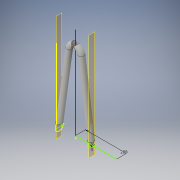
# Autodesk Inventor part: upper_arm_001
Saved by Autodesk Inventor 2016 SP1 (Build 200210100, 210)
## iProperties
Created: 2016-06-15
Part Number: upper_arm_001
Material: Generic
Document SubType Name: Modeling
Designer: asvsf
Density: 1 g/cm^3
Appearance: Default
Author: asvsf
Autodesk Inventor part; units mm, degrees
ref_plane "XZ Plane" through (0, 0, 0) normal (0, 1, 0) x (-1, 0, 0)
ref_plane "XY Plane" through (0, 0, 0) normal (0, 0, 1) x (1, 0, 0)
sketch "Sketch1" plane through (0, 0, 0) normal (0, 1, 0) x (-1, 0, 0)
  line L0 (-80, 0) -> (-30, 356.5109)
  line L1 (0, 0) -> (0, 520.9194)
  line L2 (80, 0) -> (30, 356.5109)
  arc A0 (30, 356.5109) -> (-30, 356.5109) centre (0, 352.3034) ccw
  dimension "d66" = 360
  dimension "d67" = 80
  dimension "d68" = 60
  dimension "d71" = 80
  constraints: 6 end point, 2 point on circle, 2 symmetric about line, 2 tangent, 1 centre point, 1 vertical
  measures "d66" distance of L0.start L0.end
  measures "d67" distance of L1.start L0.start
  measures "d68" distance of L2.end L0.end
  measures "d71" distance of L1.start L2.start
sketch "Sketch8" plane through (0, 0, 0) normal (0, 1, 0) x (-1, 0, 0)
  line L0 (0, 0) -> (0, 447.7409)
  constraints: 2 end point, 1 vertical
sketch "Sketch15" plane through (0, 0, 0) normal (1, 0, 0) x (0, 1, 0)
  line L0 (0, 0) -> (0, 447.7409) projected
  ellipse E0 centre (0, 0) end of major axis (13, 0) minor radius 2.8889 projected
  circle A0 centre (0, -17.1111) radius 20
  line L1 (0, 2.8889) -> (0, 11.2074)
  line L2 (0, 2.8889) -> (0, 15.4225)
  dimension "d60" = 40
  constraints: 4 end point, 2 coincident, 2 point on line, 2 vertical alignment, 1 vertical, 3 other
ref_plane "Work Plane6" through (80, 0, 0) normal (-0.1388889, 0, 0.990308) x (0, -1, 0)
sketch "Sketch16" plane through (80, 0, 0) normal (-0.1388889, 0, 0.990308) x (0, -1, 0)
  circle A0 centre (0, 0) radius 13
  point P0 (0, -79.2246)
  dimension "d72" = 26
  constraints: 1 centre point
  measures "d72" diameter of A0
sweep "Sweep5" add profiles "Sketch16" path "Sketch1" path curves L0 A0 L2
extrude "Extrusion8" [suppressed]
sketch "Sketch17" plane through (0, 0, 0) normal (0, 0, 1) x (1, 0, 0)
  line L0 (-30, -13) -> (30, -13) projected
  circle A0 centre (0, 0) radius 14
  dimension "d81" = 28
  constraints: 1 centre point
  measures "d81" diameter of A0
extrude "Extrusion9" cut sketch "Sketch17" along normal through all
sketch "Sketch18" plane through (0, 0, 0) normal (1, 0, 0) x (0, 1, 0)
  circle A0 centre (0, 0) radius 20
  ellipse E0 centre (0, 0) end of major axis (13, 0) minor radius 1.8056 projected
  dimension "d86" = 40
  constraints: 1 centre point, 1 coincident, 1 other
  measures "d86" diameter of A0
extrude "Extrusion10" cut sketch "Sketch18" along normal through all both and the other way through all contours A0 | E0
sketch "Sketch20" plane through (0, 0, 0) normal (0, 0, 1) x (1, 0, 0)
  line L0 (0, 0) -> (200, 0)
  point P0 (80, 0)
  dimension "d94" = 200
  constraints: 2 end point, 1 horizontal
  measures "d94" distance of L0.start L0.end
ref_plane "Work Plane7" through (80, 0, 0) normal (1, 0, 0) x (0, 1, 0)
sketch "Sketch22" plane through (80, 0, 0) normal (1, 0, 0) x (0, 1, 0)
  line L0 (0, 0) -> (0, -24.8938)
  constraints: 2 end point, 1 vertical
ref_plane "Work Plane8" through (-80, 0, 0) normal (1, 0, 0) x (0, 1, 0)
sketch "Sketch23" plane through (-80, 0, 0) normal (1, 0, 0) x (0, 1, 0)
  line L0 (-13, 356.5109) -> (-13, 15.1987) projected
  line L1 (-13, -2.9958) -> (30.9881, -2.9958)
  circle A0 centre (0, 0) radius 20 projected
  line L2 (0, 0) -> (0, 0)
  constraints: 4 end point, 1 perpendicular, 1 point on line, 1 vertical, 1 other
body "Solid4"
